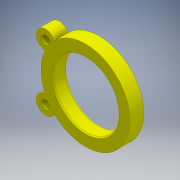
# Autodesk Inventor part: Manovella
Saved by Autodesk Inventor 2016 (Build 200138000, 138)
## iProperties
Created: 2016-09-10
Part Number: Manovella
Material: Generic
Document SubType Name: Modeling
Designer: Muhammad
Density: 1 g/cm^3
Appearance: Default
Author: Muhammad
Autodesk Inventor part; units mm, degrees
ref_plane "YZ Plane" through (0, 0, 0) normal (1, 0, 0) x (0, 1, 0)
ref_plane "XZ Plane" through (0, 0, 0) normal (0, 1, 0) x (-1, 0, 0)
ref_plane "XY Plane" through (0, 0, 0) normal (0, 0, 1) x (1, 0, 0)
sketch "Sketch1" plane through (0, 0, 0) normal (0, 1, 0) x (-1, 0, 0)
  circle A0 centre (0, 0) radius 19
  arc A1 (21.049, -15.2624) -> (21.5116, -14.6031) centre (23.3, -16.35) ccw
  arc A2 (21.5116, 14.6031) -> (21.049, 15.2624) centre (23.3, 16.35) ccw
  arc A3 (23.6235, 10.8595) -> (18.2469, 18.5216) centre (23.3, 16.35) ccw
  arc A4 (18.2469, -18.5216) -> (23.6235, -10.8595) centre (23.3, -16.35) ccw
  arc A5 (21.5116, 14.6031) -> (21.049, 15.2624) centre (0, 0) ccw
  arc A6 (18.2469, 18.5216) -> (18.2469, -18.5216) centre (0, 0) ccw
  arc A7 (21.049, -15.2624) -> (21.5116, -14.6031) centre (0, 0) ccw
  arc A8 (23.6235, -10.8595) -> (23.6235, 10.8595) centre (0, 0) ccw
  dimension "d1" = 38
  constraints: 16 point on circle, 9 centre point, 4 coincident
  measures "d1" diameter of A0
extrude "Extrusion1" add sketch "Sketch1" along normal blind 8
fillet "Fillet1" radius 0.75 2 edges at (19, 8, 0) (19, 0, 0)
body "Solid1"
